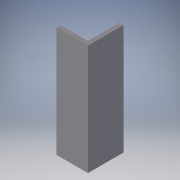
# Autodesk Inventor part: Winch Upright Bracket
Saved by Autodesk Inventor 2016 (Build 200138000, 138)
## iProperties
Created: 2015-12-16
Part Number: Winch Upright Bracket
Material: Generic
Document SubType Name: Modeling
Designer: Julia
Density: 1 g/cm^3
Appearance: Default
Author: Julia
Autodesk Inventor part; units mm, degrees
ref_plane "YZ Plane" through (0, 0, 0) normal (1, 0, 0) x (0, 1, 0)
ref_plane "XZ Plane" through (0, 0, 0) normal (0, 1, 0) x (-1, 0, 0)
ref_plane "XY Plane" through (0, 0, 0) normal (0, 0, 1) x (1, 0, 0)
sketch "Sketch1" plane through (0, 0, 0) normal (0, 1, 0) x (-1, 0, 0)
  line L0 (0, 0) -> (0, -25.4)
  line L1 (0, 0) -> (0, 3.302)
  line L2 (0, 3.302) -> (25.4, 3.302)
  line L3 (25.4, 3.302) -> (25.4, 0)
  line L4 (0, -25.4) -> (3.302, -25.4)
  line L5 (3.302, -25.4) -> (3.302, 0)
  line L6 (3.302, 0) -> (25.4, 0)
  dimension "d0" = 25.4
  dimension "d1" = 3.302
  dimension "d2" = 25.4
  dimension "d3" = 3.302
  constraints: 14 end point, 4 perpendicular, 2 vertical, 1 horizontal
  measures "d0" distance of L0.start L0.end
  measures "d1" distance of L0.start L1.end
  measures "d2" distance of L1.end L2.end
  measures "d3" distance of L0.end L4.end
extrude "Extrusion1" add sketch "Sketch1" along normal blind 88.9
body "Solid1"
